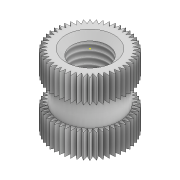
# Autodesk Inventor part: Втулка_1
Saved by Autodesk Inventor 2021.2 (Build 252289000, 289)
## iProperties
Created: 2023-04-09
Part Number: Втулка_1
Material: Типовые
Document SubType Name: Modeling
Designer: Egor
Density: 1 g/cm^3
Appearance: По умолчанию
Author: Egor
Autodesk Inventor part; units mm, degrees
ref_plane "YZ Plane" through (0, 0, 0) normal (1, 0, 0) x (0, 1, 0)
ref_plane "XZ Plane" through (0, 0, 0) normal (0, 1, 0) x (-1, 0, 0)
sketch "Эскиз1" plane through (0, 0, 0) normal (0, 1, 0) x (-1, 0, 0)
  circle A0 centre (0, 0) radius 2.5
  dimension "d0" = 5
  constraints: 1 centre point, 1 coincident
  measures "d0" diameter of A0
extrude "Выдавливание1" add sketch "Эскиз1" along normal blind 6
sketch "Эскиз2" plane through (0, 6, 0) normal (0, 1, 0) x (1, 0, 0)
  circle A0 centre (0, 0) radius 1.25
  dimension "d3" = 2.5
  constraints: 1 centre point, 1 coincident
  measures "d3" diameter of A0
hole "Отверстие1" at (0, 6, 0) direction (0, -1, 0) diameter 2.5 depth 12
thread "Резьба1" size "M3x0.5" class "6H" standard "ANSI Metric M Profile" full length
sketch "Эскиз3" plane through (0, 6, 0) normal (0, 1, 0) x (1, 0, 0)
  circle A0 centre (0, 0) radius 2.5 projected
  line L0 (-2.5, 0) -> (-3, 0)
  line L1 (-3, 0) -> (-2.0603, 0.342)
  line L2 (-3, 0) -> (-2.054, 0) construction
  line L3 (-3, 0) -> (-2.0766, -0.3361)
  line L4 (-3, 0) -> (-2.0173, 0) construction
  line L5 (-2.4786, -0.3263) -> (-2.9743, -0.3916)
  line L6 (-2.9743, -0.3916) -> (-2.0873, 0.0702)
  line L7 (-2.9743, -0.3916) -> (-2.0364, -0.2681) construction
  line L8 (-2.9743, -0.3916) -> (-2.015, -0.6043)
  line L9 (-2.9743, -0.3916) -> (-2.0001, -0.2633) construction
  line L10 (-2.4148, -0.647) -> (-2.8978, -0.7765)
  line L11 (-2.8978, -0.7765) -> (-2.0786, -0.2029)
  line L12 (-2.8978, -0.7765) -> (-1.984, -0.5316) construction
  line L13 (-2.8978, -0.7765) -> (-1.9188, -0.8621)
  line L14 (-2.8978, -0.7765) -> (-1.9486, -0.5221) construction
  line L15 (-2.3097, -0.9567) -> (-2.7716, -1.1481)
  line L16 (-2.7716, -1.1481) -> (-2.0344, -0.4725)
  line L17 (-2.7716, -1.1481) -> (-1.8977, -0.786) construction
  line L18 (-2.7716, -1.1481) -> (-1.7899, -1.1052)
  line L19 (-2.7716, -1.1481) -> (-1.8638, -0.772) construction
  line L20 (-2.1651, -1.25) -> (-2.5981, -1.5)
  line L21 (-2.5981, -1.5) -> (-1.9553, -0.734)
  line L22 (-2.5981, -1.5) -> (-1.7788, -1.027) construction
  line L23 (-2.5981, -1.5) -> (-1.6303, -1.3294)
  line L24 (-2.5981, -1.5) -> (-1.7471, -1.0087) construction
  line L25 (-1.9834, -1.5219) -> (-2.3801, -1.8263)
  line L26 (-2.3801, -1.8263) -> (-1.8428, -0.9829)
  line L27 (-2.3801, -1.8263) -> (-1.6296, -1.2504) construction
  line L28 (-2.3801, -1.8263) -> (-1.4429, -1.5308)
  line L29 (-2.3801, -1.8263) -> (-1.6005, -1.2281) construction
  line L30 (-1.7678, -1.7678) -> (-2.1213, -2.1213)
  line L31 (-2.1213, -2.1213) -> (-1.6987, -1.215)
  line L32 (-2.1213, -2.1213) -> (-1.4524, -1.4524) construction
  line L33 (-2.1213, -2.1213) -> (-1.2307, -1.706)
  line L34 (-2.1213, -2.1213) -> (-1.4265, -1.4265) construction
  line L35 (-1.5219, -1.9834) -> (-1.8263, -2.3801)
  line L36 (-1.8263, -2.3801) -> (-1.5256, -1.4263)
  line L37 (-1.8263, -2.3801) -> (-1.2504, -1.6296) construction
  line L38 (-1.8263, -2.3801) -> (-0.9975, -1.8521)
  line L39 (-1.8263, -2.3801) -> (-1.2281, -1.6005) construction
  line L40 (-1.25, -2.1651) -> (-1.5, -2.5981)
  line L41 (-1.5, -2.5981) -> (-1.3264, -1.6133)
  line L42 (-1.5, -2.5981) -> (-1.027, -1.7788) construction
  line L43 (-1.5, -2.5981) -> (-0.7472, -1.9664)
  line L44 (-1.5, -2.5981) -> (-1.0087, -1.7471) construction
  line L45 (-0.9567, -2.3097) -> (-1.1481, -2.7716)
  line L46 (-1.1481, -2.7716) -> (-1.1044, -1.7726)
  line L47 (-1.1481, -2.7716) -> (-0.786, -1.8977) construction
  line L48 (-1.1481, -2.7716) -> (-0.4842, -2.0471)
  line L49 (-1.1481, -2.7716) -> (-0.772, -1.8638) construction
  line L50 (-0.647, -2.4148) -> (-0.7765, -2.8978)
  line L51 (-0.7765, -2.8978) -> (-0.8636, -1.9016)
  line L52 (-0.7765, -2.8978) -> (-0.5316, -1.984) construction
  line L53 (-0.7765, -2.8978) -> (-0.2128, -2.0928)
  line L54 (-0.7765, -2.8978) -> (-0.5221, -1.9486) construction
  line L55 (-0.3263, -2.4786) -> (-0.3916, -2.9743)
  line L56 (-0.3916, -2.9743) -> (-0.608, -1.998)
  line L57 (-0.3916, -2.9743) -> (-0.2681, -2.0364) construction
  line L58 (-0.3916, -2.9743) -> (0.0622, -2.1027)
  line L59 (-0.3916, -2.9743) -> (-0.2633, -2.0001) construction
  line L60 (0, -2.5) -> (0, -3)
  line L61 (0, -3) -> (-0.342, -2.0603)
  line L62 (0, -3) -> (0, -2.054) construction
  line L63 (0, -3) -> (0.3361, -2.0766)
  line L64 (0, -3) -> (0, -2.0173) construction
  line L65 (0.3263, -2.4786) -> (0.3916, -2.9743)
  line L66 (0.3916, -2.9743) -> (-0.0702, -2.0873)
  line L67 (0.3916, -2.9743) -> (0.2681, -2.0364) construction
  line L68 (0.3916, -2.9743) -> (0.6043, -2.015)
  line L69 (0.3916, -2.9743) -> (0.2633, -2.0001) construction
  line L70 (0.647, -2.4148) -> (0.7765, -2.8978)
  line L71 (0.7765, -2.8978) -> (0.2029, -2.0786)
  line L72 (0.7765, -2.8978) -> (0.5316, -1.984) construction
  line L73 (0.7765, -2.8978) -> (0.8621, -1.9188)
  line L74 (0.7765, -2.8978) -> (0.5221, -1.9486) construction
  line L75 (0.9567, -2.3097) -> (1.1481, -2.7716)
  line L76 (1.1481, -2.7716) -> (0.4725, -2.0344)
  line L77 (1.1481, -2.7716) -> (0.786, -1.8977) construction
  line L78 (1.1481, -2.7716) -> (1.1052, -1.7899)
  line L79 (1.1481, -2.7716) -> (0.772, -1.8638) construction
  line L80 (1.25, -2.1651) -> (1.5, -2.5981)
  line L81 (1.5, -2.5981) -> (0.734, -1.9553)
  line L82 (1.5, -2.5981) -> (1.027, -1.7788) construction
  line L83 (1.5, -2.5981) -> (1.3294, -1.6303)
  line L84 (1.5, -2.5981) -> (1.0087, -1.7471) construction
  line L85 (1.5219, -1.9834) -> (1.8263, -2.3801)
  line L86 (1.8263, -2.3801) -> (0.9829, -1.8428)
  line L87 (1.8263, -2.3801) -> (1.2504, -1.6296) construction
  line L88 (1.8263, -2.3801) -> (1.5308, -1.4429)
  line L89 (1.8263, -2.3801) -> (1.2281, -1.6005) construction
  line L90 (1.7678, -1.7678) -> (2.1213, -2.1213)
  line L91 (2.1213, -2.1213) -> (1.215, -1.6987)
  line L92 (2.1213, -2.1213) -> (1.4524, -1.4524) construction
  line L93 (2.1213, -2.1213) -> (1.706, -1.2307)
  line L94 (2.1213, -2.1213) -> (1.4265, -1.4265) construction
  line L95 (1.9834, -1.5219) -> (2.3801, -1.8263)
  line L96 (2.3801, -1.8263) -> (1.4263, -1.5256)
  line L97 (2.3801, -1.8263) -> (1.6296, -1.2504) construction
  line L98 (2.3801, -1.8263) -> (1.8521, -0.9975)
  line L99 (2.3801, -1.8263) -> (1.6005, -1.2281) construction
  line L100 (2.1651, -1.25) -> (2.5981, -1.5)
  line L101 (2.5981, -1.5) -> (1.6133, -1.3264)
  line L102 (2.5981, -1.5) -> (1.7788, -1.027) construction
  line L103 (2.5981, -1.5) -> (1.9664, -0.7472)
  line L104 (2.5981, -1.5) -> (1.7471, -1.0087) construction
  line L105 (2.3097, -0.9567) -> (2.7716, -1.1481)
  line L106 (2.7716, -1.1481) -> (1.7726, -1.1044)
  line L107 (2.7716, -1.1481) -> (1.8977, -0.786) construction
  line L108 (2.7716, -1.1481) -> (2.0471, -0.4842)
  line L109 (2.7716, -1.1481) -> (1.8638, -0.772) construction
  line L110 (2.4148, -0.647) -> (2.8978, -0.7765)
  line L111 (2.8978, -0.7765) -> (1.9016, -0.8636)
  line L112 (2.8978, -0.7765) -> (1.984, -0.5316) construction
  line L113 (2.8978, -0.7765) -> (2.0928, -0.2128)
  line L114 (2.8978, -0.7765) -> (1.9486, -0.5221) construction
  line L115 (2.4786, -0.3263) -> (2.9743, -0.3916)
  line L116 (2.9743, -0.3916) -> (1.998, -0.608)
  line L117 (2.9743, -0.3916) -> (2.0364, -0.2681) construction
  line L118 (2.9743, -0.3916) -> (2.1027, 0.0622)
  line L119 (2.9743, -0.3916) -> (2.0001, -0.2633) construction
  line L120 (2.5, 0) -> (3, 0)
  line L121 (3, 0) -> (2.0603, -0.342)
  line L122 (3, 0) -> (2.054, 0) construction
  line L123 (3, 0) -> (2.0766, 0.3361)
  line L124 (3, 0) -> (2.0173, 0) construction
  line L125 (2.4786, 0.3263) -> (2.9743, 0.3916)
  line L126 (2.9743, 0.3916) -> (2.0873, -0.0702)
  line L127 (2.9743, 0.3916) -> (2.0364, 0.2681) construction
  line L128 (2.9743, 0.3916) -> (2.015, 0.6043)
  line L129 (2.9743, 0.3916) -> (2.0001, 0.2633) construction
  line L130 (2.4148, 0.647) -> (2.8978, 0.7765)
  line L131 (2.8978, 0.7765) -> (2.0786, 0.2029)
  line L132 (2.8978, 0.7765) -> (1.984, 0.5316) construction
  line L133 (2.8978, 0.7765) -> (1.9188, 0.8621)
  line L134 (2.8978, 0.7765) -> (1.9486, 0.5221) construction
  line L135 (2.3097, 0.9567) -> (2.7716, 1.1481)
  line L136 (2.7716, 1.1481) -> (2.0344, 0.4725)
  line L137 (2.7716, 1.1481) -> (1.8977, 0.786) construction
  line L138 (2.7716, 1.1481) -> (1.7899, 1.1052)
  line L139 (2.7716, 1.1481) -> (1.8638, 0.772) construction
  line L140 (2.1651, 1.25) -> (2.5981, 1.5)
  line L141 (2.5981, 1.5) -> (1.9553, 0.734)
  line L142 (2.5981, 1.5) -> (1.7788, 1.027) construction
  line L143 (2.5981, 1.5) -> (1.6303, 1.3294)
  line L144 (2.5981, 1.5) -> (1.7471, 1.0087) construction
  line L145 (1.9834, 1.5219) -> (2.3801, 1.8263)
  line L146 (2.3801, 1.8263) -> (1.8428, 0.9829)
  line L147 (2.3801, 1.8263) -> (1.6296, 1.2504) construction
  line L148 (2.3801, 1.8263) -> (1.4429, 1.5308)
  line L149 (2.3801, 1.8263) -> (1.6005, 1.2281) construction
  line L150 (1.7678, 1.7678) -> (2.1213, 2.1213)
  line L151 (2.1213, 2.1213) -> (1.6987, 1.215)
  line L152 (2.1213, 2.1213) -> (1.4524, 1.4524) construction
  line L153 (2.1213, 2.1213) -> (1.2307, 1.706)
  line L154 (2.1213, 2.1213) -> (1.4265, 1.4265) construction
  line L155 (1.5219, 1.9834) -> (1.8263, 2.3801)
  line L156 (1.8263, 2.3801) -> (1.5256, 1.4263)
  line L157 (1.8263, 2.3801) -> (1.2504, 1.6296) construction
  line L158 (1.8263, 2.3801) -> (0.9975, 1.8521)
  line L159 (1.8263, 2.3801) -> (1.2281, 1.6005) construction
  line L160 (1.25, 2.1651) -> (1.5, 2.5981)
  line L161 (1.5, 2.5981) -> (1.3264, 1.6133)
  line L162 (1.5, 2.5981) -> (1.027, 1.7788) construction
  line L163 (1.5, 2.5981) -> (0.7472, 1.9664)
  line L164 (1.5, 2.5981) -> (1.0087, 1.7471) construction
  line L165 (0.9567, 2.3097) -> (1.1481, 2.7716)
  line L166 (1.1481, 2.7716) -> (1.1044, 1.7726)
  line L167 (1.1481, 2.7716) -> (0.786, 1.8977) construction
  line L168 (1.1481, 2.7716) -> (0.4842, 2.0471)
  line L169 (1.1481, 2.7716) -> (0.772, 1.8638) construction
  line L170 (0.647, 2.4148) -> (0.7765, 2.8978)
  line L171 (0.7765, 2.8978) -> (0.8636, 1.9016)
  line L172 (0.7765, 2.8978) -> (0.5316, 1.984) construction
  line L173 (0.7765, 2.8978) -> (0.2128, 2.0928)
  line L174 (0.7765, 2.8978) -> (0.5221, 1.9486) construction
  line L175 (0.3263, 2.4786) -> (0.3916, 2.9743)
  line L176 (0.3916, 2.9743) -> (0.608, 1.998)
  line L177 (0.3916, 2.9743) -> (0.2681, 2.0364) construction
  line L178 (0.3916, 2.9743) -> (-0.0622, 2.1027)
  line L179 (0.3916, 2.9743) -> (0.2633, 2.0001) construction
  line L180 (0, 2.5) -> (0, 3)
  line L181 (0, 3) -> (0.342, 2.0603)
  line L182 (0, 3) -> (0, 2.054) construction
  line L183 (0, 3) -> (-0.3361, 2.0766)
  line L184 (0, 3) -> (0, 2.0173) construction
  line L185 (-0.3263, 2.4786) -> (-0.3916, 2.9743)
  line L186 (-0.3916, 2.9743) -> (0.0702, 2.0873)
  line L187 (-0.3916, 2.9743) -> (-0.2681, 2.0364) construction
  line L188 (-0.3916, 2.9743) -> (-0.6043, 2.015)
  line L189 (-0.3916, 2.9743) -> (-0.2633, 2.0001) construction
  line L190 (-0.647, 2.4148) -> (-0.7765, 2.8978)
  line L191 (-0.7765, 2.8978) -> (-0.2029, 2.0786)
  line L192 (-0.7765, 2.8978) -> (-0.5316, 1.984) construction
  line L193 (-0.7765, 2.8978) -> (-0.8621, 1.9188)
  line L194 (-0.7765, 2.8978) -> (-0.5221, 1.9486) construction
  line L195 (-0.9567, 2.3097) -> (-1.1481, 2.7716)
  line L196 (-1.1481, 2.7716) -> (-0.4725, 2.0344)
  line L197 (-1.1481, 2.7716) -> (-0.786, 1.8977) construction
  line L198 (-1.1481, 2.7716) -> (-1.1052, 1.7899)
  line L199 (-1.1481, 2.7716) -> (-0.772, 1.8638) construction
  line L200 (-1.25, 2.1651) -> (-1.5, 2.5981)
  line L201 (-1.5, 2.5981) -> (-0.734, 1.9553)
  line L202 (-1.5, 2.5981) -> (-1.027, 1.7788) construction
  line L203 (-1.5, 2.5981) -> (-1.3294, 1.6303)
  line L204 (-1.5, 2.5981) -> (-1.0087, 1.7471) construction
  line L205 (-1.5219, 1.9834) -> (-1.8263, 2.3801)
  line L206 (-1.8263, 2.3801) -> (-0.9829, 1.8428)
  line L207 (-1.8263, 2.3801) -> (-1.2504, 1.6296) construction
  line L208 (-1.8263, 2.3801) -> (-1.5308, 1.4429)
  line L209 (-1.8263, 2.3801) -> (-1.2281, 1.6005) construction
  line L210 (-1.7678, 1.7678) -> (-2.1213, 2.1213)
  line L211 (-2.1213, 2.1213) -> (-1.215, 1.6987)
  line L212 (-2.1213, 2.1213) -> (-1.4524, 1.4524) construction
  line L213 (-2.1213, 2.1213) -> (-1.706, 1.2307)
  line L214 (-2.1213, 2.1213) -> (-1.4265, 1.4265) construction
  line L215 (-1.9834, 1.5219) -> (-2.3801, 1.8263)
  line L216 (-2.3801, 1.8263) -> (-1.4263, 1.5256)
  line L217 (-2.3801, 1.8263) -> (-1.6296, 1.2504) construction
  line L218 (-2.3801, 1.8263) -> (-1.8521, 0.9975)
  line L219 (-2.3801, 1.8263) -> (-1.6005, 1.2281) construction
  line L220 (-2.1651, 1.25) -> (-2.5981, 1.5)
  line L221 (-2.5981, 1.5) -> (-1.6133, 1.3264)
  line L222 (-2.5981, 1.5) -> (-1.7788, 1.027) construction
  line L223 (-2.5981, 1.5) -> (-1.9664, 0.7472)
  line L224 (-2.5981, 1.5) -> (-1.7471, 1.0087) construction
  line L225 (-2.3097, 0.9567) -> (-2.7716, 1.1481)
  line L226 (-2.7716, 1.1481) -> (-1.7726, 1.1044)
  line L227 (-2.7716, 1.1481) -> (-1.8977, 0.786) construction
  line L228 (-2.7716, 1.1481) -> (-2.0471, 0.4842)
  line L229 (-2.7716, 1.1481) -> (-1.8638, 0.772) construction
  line L230 (-2.4148, 0.647) -> (-2.8978, 0.7765)
  line L231 (-2.8978, 0.7765) -> (-1.9016, 0.8636)
  line L232 (-2.8978, 0.7765) -> (-1.984, 0.5316) construction
  line L233 (-2.8978, 0.7765) -> (-2.0928, 0.2128)
  line L234 (-2.8978, 0.7765) -> (-1.9486, 0.5221) construction
  line L235 (-2.4786, 0.3263) -> (-2.9743, 0.3916)
  line L236 (-2.9743, 0.3916) -> (-1.998, 0.608)
  line L237 (-2.9743, 0.3916) -> (-2.0364, 0.2681) construction
  line L238 (-2.9743, 0.3916) -> (-2.1027, -0.0622)
  line L239 (-2.9743, 0.3916) -> (-2.0001, 0.2633) construction
  point P0 (-2.5422, -0.1666)
  point P1 (-2.4987, -0.497)
  point P2 (-2.4125, -0.8189)
  point P3 (-2.2849, -1.1268)
  point P4 (-2.1183, -1.4154)
  point P5 (-1.9154, -1.6798)
  point P6 (-1.6798, -1.9154)
  point P7 (-1.4154, -2.1183)
  point P8 (-1.1268, -2.2849)
  point P9 (-0.8189, -2.4125)
  point P10 (-0.497, -2.4987)
  point P11 (-0.1666, -2.5422)
  point P12 (0.1666, -2.5422)
  point P13 (0.497, -2.4987)
  point P14 (0.8189, -2.4125)
  point P15 (1.1268, -2.2849)
  point P16 (1.4154, -2.1183)
  point P17 (1.6798, -1.9154)
  point P18 (1.9154, -1.6798)
  point P19 (2.1183, -1.4154)
  point P20 (2.2849, -1.1268)
  point P21 (2.4125, -0.8189)
  point P22 (2.4987, -0.497)
  point P23 (2.5422, -0.1666)
  point P24 (2.5422, 0.1666)
  point P25 (2.4987, 0.497)
  point P26 (2.4125, 0.8189)
  point P27 (2.2849, 1.1268)
  point P28 (2.1183, 1.4154)
  point P29 (1.9154, 1.6798)
  point P30 (1.6798, 1.9154)
  point P31 (1.4154, 2.1183)
  point P32 (1.1268, 2.2849)
  point P33 (0.8189, 2.4125)
  point P34 (0.497, 2.4987)
  point P35 (0.1666, 2.5422)
  point P36 (-0.1666, 2.5422)
  point P37 (-0.497, 2.4987)
  point P38 (-0.8189, 2.4125)
  point P39 (-1.1268, 2.2849)
  point P40 (-1.4154, 2.1183)
  point P41 (-1.6798, 1.9154)
  point P42 (-1.9154, 1.6798)
  point P43 (-2.1183, 1.4154)
  point P44 (-2.2849, 1.1268)
  point P45 (-2.4125, 0.8189)
  point P46 (-2.4987, 0.497)
  point P47 (-2.5422, 0.1666)
  dimension "d13" = 0.5
  dimension "d14" = 1
  dimension "d15" = 20
  dimension "d17" = 20
  dimension "d20" = 360
  constraints: 480 end point, 3 horizontal, 1 equal length, 1 horizontal alignment, 530 other
  measures "d13" distance of L0.start L0.end
  measures "d14" distance of L0.end L1.end
  measures "d15" angle of L0 L1
  measures "d17" angle of L3 L4
extrude "Выдавливание2" add sketch "Эскиз3" against normal blind 6
sketch "Эскиз4" plane through (0, 6, 0) normal (0, 1, 0) x (1, 0, 0)
  circle A0 centre (0, 0) radius 1.25
  dimension "d24" = 2.5
  constraints: 1 centre point, 1 coincident
  measures "d24" diameter of A0
hole "Отверстие2" at (0, 6, 0) direction (0, -1, 0) diameter 3 depth 12
thread "Резьба2" size "M3x0.5" class "6H" standard "ANSI Metric M Profile" full length
sketch "Эскиз5" plane through (0, 6, 0) normal (0, 1, 0) x (1, 0, 0)
  point P0 (0, 0)
sketch "Эскиз6" plane through (0, 6, 0) normal (0, 1, 0) x (1, 0, 0)
  point P0 (0, 0)
ref_plane "РабПлоскость1" through (0, 4, 0) normal (0, 1, 0) x (1, 0, 0)
sketch "Эскиз7" plane through (0, 4, 0) normal (0, 1, 0) x (1, 0, 0)
  circle A0 centre (0, 0) radius 2.5
  circle A1 centre (0, 0) radius 4.2127
  dimension "d35" = 5
  constraints: 2 centre point, 2 coincident
  measures "d35" diameter of A0
extrude "Выдавливание3" cut sketch "Эскиз7" against normal blind 2
sketch "Эскиз8" plane through (0, 6, 0) normal (0, 1, 0) x (1, 0, 0)
  point P0 (0, 0)
chamfer "Фаска1" distance 0.5 angle 45 2 edges at (0, 6, -1.5) (0, 0, -1.5)
sketch "Эскиз9" plane through (0, 6, 0) normal (0, 1, 0) x (1, 0, 0)
  point P0 (0, 0)
